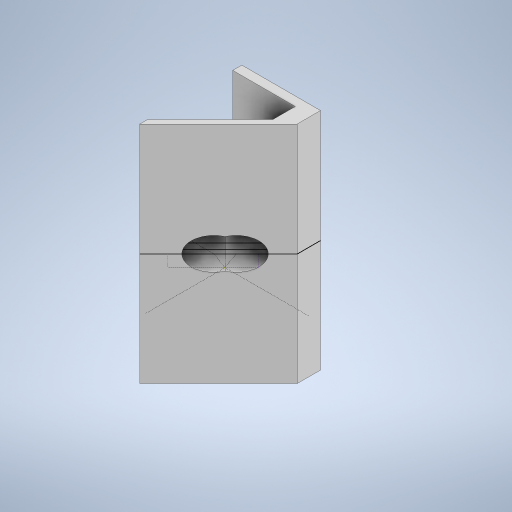
# Autodesk Inventor part: round dichroic holder
Saved by Autodesk Inventor 2024 (Build 280153000, 153)
## iProperties
Created: 2024-11-13
Part Number: round dichroic holder
Material: Generic
Document SubType Name: Modeling
Designer: Williamow
Density: 1 g/cm^3
Appearance: Default
Author: Williamow
Autodesk Inventor part; units mm, degrees
ref_plane "YZ Plane" through (0, 0, 0) normal (1, 0, 0) x (0, 1, 0)
ref_plane "XZ Plane" through (0, 0, 0) normal (0, 1, 0) x (-1, 0, 0)
ref_plane "XY Plane" through (0, 0, 0) normal (0, 0, 1) x (1, 0, 0)
sketch "Sketch9" plane through (0, 0, 0) normal (0, 1, 0) x (-1, 0, 0)
  line L0 (3.4, -4.445) -> (-1.5, -4.445)
  line L1 (-0.3017, -1.7866) -> (-1.0442, -1.0442) construction
  line L2 (-1.0442, -1.0442) -> (1.7843, 1.7843) construction
  line L3 (1.7843, 1.7843) -> (2.5267, 1.0418) construction
  line L4 (0, 0) -> (0, 4.9841) construction
  line L5 (0, 0) -> (-5.2239, 0) construction
  line L6 (0, 0) -> (1.0887, -0.3962) construction
  line L7 (1.0887, -0.3962) -> (3.6157, -0.3962) construction
  line L8 (-0.3017, -1.7866) -> (2.5267, 1.0418) construction
  line L9 (3.4, 1.9151) -> (-1.5, -2.9849)
  line L10 (-1.5, -2.9849) -> (-1.5, -4.445)
  line L11 (-0.5, -2.494) -> (-0.5, -3.8793)
  line L12 (-0.5, -3.8793) -> (3.4, -3.8793)
  line L13 (3.4, -3.8793) -> (3.4, -4.445)
  line L14 (3.4, -3.8793) -> (2.8343, -4.445) construction
  line L15 (3.4, 1.9151) -> (3.4, 1.406)
  line L16 (3.4, 1.406) -> (-0.5, -2.494)
  line L17 (0, 0) -> (0.5624, -0.5624) construction
  line L18 (3.4, 1.406) -> (3.4, 0.7133)
  line L19 (3.4, 0.7133) -> (-0.5, -3.1867)
  line L20 (3.4, 0.7133) -> (3.4, -3.8793)
  line L21 (0, 0) -> (0.3962, -1.0887) construction
  dimension "d82" = 1.05
  dimension "d83" = 4.445
  dimension "d84" = 3.4
  dimension "d86" = 4
  dimension "d102" = 135
  dimension "d104" = 1
  dimension "d115" = 45
  dimension "d116" = 0.8
  dimension "d125" = 1.5
  dimension "d126" = 0.36
  dimension "d127" = 25
  dimension "d133" = 25
  constraints: 44 end point, 5 perpendicular, 4 parallel, 4 point on line, 4 vertical, 3 horizontal, 2 collinear, 1 coincident, 1 midpoint, 1 vertical alignment
  measures "d82" distance of L2.end L3.end
  measures "d83" distance from line of L5 L0.end
  measures "d84" distance from line of L0.start L4
  measures "d86" distance of L1.end L2.end
  measures "d102" angle of L9 L10
  measures "d104" distance between parallel lines of L10 L11
  measures "d115" angle of L13 L14
  measures "d116" distance of L12.end L14.end
  measures "d125" horizontal distance of L0.end point (0, 0)
  measures "d126" distance between parallel lines of L16 L9
  measures "d127" angle of L6 L17
  measures "d133" angle of L21 L17
sketch "Sketch14" plane through (0, 0, 0) normal (0, 1, 0) x (-1, 0, 0)
  line L0 (0, 0) -> (0.3962, -1.0887) construction
  line L1 (0, 0) -> (1.0887, -0.3962) construction
  line L2 (0.3962, 3.3492) -> (1.3962, 3.3492)
  line L3 (1.3962, 3.3492) -> (1.3962, -4.9901)
  line L4 (1.3962, -4.9901) -> (0.3962, -4.9901)
  line L5 (0.3962, -4.9901) -> (0.3962, 3.3492)
  line L6 (-1.8344, -0.3962) -> (3.8418, -0.3962)
  line L7 (3.8418, -0.3962) -> (3.8418, -1.3962)
  line L8 (3.8418, -1.3962) -> (-1.8344, -1.3962)
  line L9 (-1.8344, -1.3962) -> (-1.8344, -0.3962)
  dimension "d134" = 1
  constraints: 16 end point, 4 parallel, 3 perpendicular, 2 horizontal, 2 point on line
  measures "d134" distance of L3.end L4.end
extrude "Extrusion14" add sketch "Sketch9" along normal mid plane 14 contours L0 L10 L9 L15 L16 L11 L12 L13
sketch "Sketch13" plane through (-3.4, -7, -3.8793) normal (-1, 0, 0) x (0, 0, 1)
  line L0 (0, 0) -> (0, 14) projected
  line L1 (0, 8.6843) -> (0, 11.3157)
  line L2 (0, 11.3157) -> (0.5657, 10.75)
  line L3 (0.5657, 10.75) -> (0.5657, 9.25)
  line L4 (0.5657, 9.25) -> (0, 8.6843)
  line L5 (0, 7) -> (-0.5657, 7) projected
  line L6 (-0.5657, 14) -> (0, 14) projected
  line L7 (0.5657, 10) -> (0, 10) construction
  line L8 (0, 2.6843) -> (0.5657, 3.25)
  line L9 (0.5657, 3.25) -> (0.5657, 4.75)
  line L10 (0.5657, 4.75) -> (0, 5.3157)
  point P0 (3.8793, 7)
  point P1 (-0.2828, 7)
  dimension "d117" = 45
  dimension "d118" = 3
  dimension "d119" = 1.5
  constraints: 16 end point, 4 symmetric about line, 3 midpoint, 2 equal length, 1 horizontal, 1 horizontal alignment, 1 parallel, 1 point on line, 1 vertical
  measures "d117" angle of L0 L4
  measures "d118" vertical distance of L7.end point (-0.283, 7)
  measures "d119" distance of L2.end L3.end
extrude "Extrusion16" add sketch "Sketch13" against normal up to next
sketch "Sketch12" plane through (1.5, 7, -4.445) normal (0, 0, -1) x (-1, 0, 0)
  circle A0 centre (3, -4) radius 0.6
  circle A1 centre (3, -10) radius 0.6
  point P0 (1.5, -7)
  dimension "d109" = 1.5
  dimension "d110" = 3
  dimension "d111" = 3
  dimension "d112" = 1.2
  constraints: 2 centre point, 1 equal radius, 1 vertical alignment
  measures "d109" horizontal distance of point (1.5, -7) A0.centre
  measures "d110" vertical distance of point (1.5, -7) A0.centre
  measures "d111" vertical distance of A1.centre point (1.5, -7)
  measures "d112" diameter of A1
extrude "Extrusion15" cut sketch "Sketch12" against normal blind 2
extrude "Extrusion17" add sketch "Sketch9" along normal mid plane 3.6 contours L12 L11 L19 L20 | L19 L11 L16 L18
revolve "Revolution5" cut sketch "Sketch14" angle 360 about axis through (-0.3962, 0, -4.9901) along (0, 0, 1) contours L2 L3 L6 L5 | L6 L3 L8 L5 | L8 L3 L4 L5
revolve "Revolution6" cut sketch "Sketch14" angle 360 about axis through (1.8344, 0, -0.3962) along (-1, 0, 0) contours L6 L3 L8 L5 | L5 L8 L9 L6 | L6 L7 L8 L3
body "Solid1"
body "Solid5"
